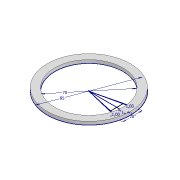
# Autodesk Inventor part: NeoPixel-24
Saved by Autodesk Inventor 2020.3 (Build 243373000, 373)
## iProperties
Created: 2021-08-28
Part Number: NeoPixel-24
Material: Generic
Document SubType Name: Modeling
Designer: Yusuf
Mass: 5.60885 g
Surface Area: 53.2311 cm^2
Volume: 5.60885 cm^3
Density: 1 g/cm^3
Appearance: Default
Author: Yusuf
Autodesk Inventor part; units mm, degrees
ref_plane "YZ Plane" through (0, 0, 0) normal (1, 0, 0) x (0, 1, 0)
ref_plane "XZ Plane" through (0, 0, 0) normal (0, 1, 0) x (-1, 0, 0)
ref_plane "XY Plane" through (0, 0, 0) normal (0, 0, 1) x (1, 0, 0)
sketch "Sketch1" plane through (0, 0, 0) normal (0, 1, 0) x (-1, 0, 0)
  circle A0 centre (0, 0) radius 42.5
  circle A1 centre (0, 0) radius 35
  line L0 (0, 0) -> (-41.3068, 10)
  line L1 (0, 0) -> (-41.3068, -10)
  line L2 (0, 0) -> (-42.5, 0)
  line L3 (-28.5133, 6.9028) -> (-28.5133, -6.9028)
  arc A2 (-34.9893, 8.4706) -> (-34.9893, -8.4706) centre (0, 0) ccw
  arc A3 (-40.3349, 9.7647) -> (-40.3349, -9.7647) centre (0, 0) ccw
  line L4 (0, 0) -> (-41.475, 9.2776)
  line L5 (0, 0) -> (-41.475, -9.2776)
  point P0 (-28.5133, 0)
  point P1 (-40.4991, -9.0593)
  point P2 (-35.1318, -7.8587)
  point P3 (-35.1318, 7.8587)
  point P4 (-40.4991, 9.0593)
  dimension "d0" = 85
  dimension "d1" = 70
  dimension "d2" = 20
  dimension "d4" = 1
  dimension "d5" = 1
  dimension "d6" = 1
  dimension "d7" = 1
  constraints: 12 end point, 9 point on circle, 6 point on line, 4 centre point, 4 coincident, 1 horizontal, 1 horizontal alignment, 1 midpoint, 1 vertical
  measures "d0" diameter of A0
  measures "d1" diameter of A1
  measures "d2" distance of L1.end L0.end
  measures "d4" radial gap between concentric circles of A2 A1
  measures "d5" radial gap between concentric circles of A0 A3
  measures "d6" angle of L0 L4
  measures "d7" angle of L1 L5
extrude "Extrusion1" add sketch "Sketch1" along normal blind 3.2 contours A0 L1 A1 L0 | L0 A3 L4 A0 | A0 L5 A3 L1 | L4 A3 L2 A0 | L0 A2 L4 A3 | A0 L2 A3 L5 | A3 L5 A2 L1 | L4 A2 L2 A3 | L0 A1 L4 A2 | A3 L2 A2 L5 | A2 L5 A1 L1 | L4 A1 L2 A2 | A2 L2 A1 L5
extrude "Extrusion2" cut sketch "Sketch1" along normal blind 2.5 contours L4 A2 L2 A3 | A3 L2 A2 L5
body "Solid1"
